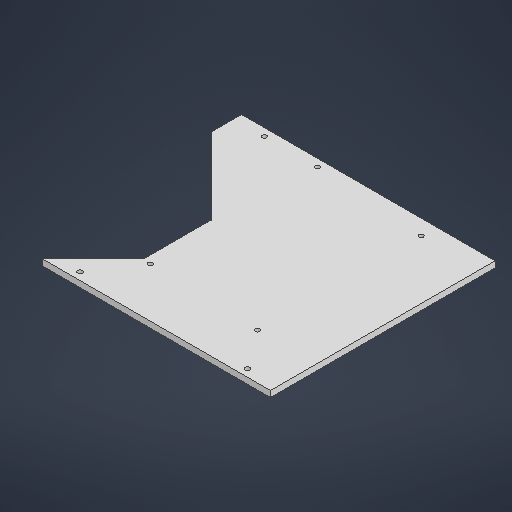
# Autodesk Inventor part: SidePlate_Ebox
Saved by Autodesk Inventor 2025.1 (Build 291241000, 241)
## iProperties
Created: 2025-03-19
Part Number: SidePlate_Ebox
Material: Generic
Document SubType Name: Modeling
Designer: m_kni
Density: 1 g/cm^3
Appearance: Default
Author: m_kni
Autodesk Inventor part; units mm, degrees
ref_plane "YZ Plane" through (0, 0, 0) normal (1, 0, 0) x (0, 1, 0)
ref_plane "XZ Plane" through (0, 0, 0) normal (0, 1, 0) x (-1, 0, 0)
ref_plane "XY Plane" through (0, 0, 0) normal (0, 0, 1) x (1, 0, 0)
sketch "Sketch1" plane through (0, 0, 0) normal (0, 1, 0) x (-1, 0, 0)
  line L0 (-83.0918, 73.8924) -> (-83.0918, -73.6076)
  line L1 (-83.0918, 73.8924) -> (-83.0918, -73.6076)
  line L2 (66.9082, 73.8924) -> (-83.0918, 73.8924)
  line L3 (-83.0918, 73.8924) -> (-83.0918, -73.6076)
  line L4 (-83.0918, -73.6076) -> (83.4082, -73.6076)
  line L5 (83.4082, -73.6076) -> (83.4082, -53.6076)
  line L6 (83.4082, -53.6076) -> (33.4082, -3.6076)
  line L7 (33.4082, -3.6076) -> (33.4082, 40.3924)
  line L8 (33.4082, 40.3924) -> (66.9082, 73.8924)
  point P0 (0, 0)
  point P1 (-8.0918, 73.8924)
  constraints: 18 end point, 1 vertical
extrude "Extrusion1" add sketch "Sketch1" along normal blind 4
sketch "Sketch2" plane through (0, 4, 0) normal (0, 1, 0) x (1, 0, 0)
  line L0 (83.0918, -73.8924) -> (83.0918, 73.6076) projected
  line L1 (-66.9082, -73.8924) -> (83.0918, -73.8924) projected
  line L2 (83.0918, -73.8924) -> (-66.9082, -73.8924)
  circle A0 centre (-46.9082, -68.8924) radius 1.6
  circle A1 centre (63.0918, -68.8924) radius 1.6
  point P0 (0, 0)
  dimension "d2" = 20
  dimension "d3" = 5
  dimension "d4" = 20
  dimension "d5" = 3.2
  dimension "d6" = 3.2
  constraints: 2 centre point, 2 coincident, 2 end point, 1 collinear
  measures "d2" horizontal distance of point (-46.908, -68.892) L1.start
  measures "d3" distance from line of L1 point (-46.908, -68.892)
  measures "d4" distance from line of point (63.092, -68.892) L0
  measures "d5" diameter of A0
  measures "d6" diameter of A1
extrude "Extrusion2" cut sketch "Sketch2" against normal blind 10
sketch "Sketch3" plane through (0, 4, 0) normal (0, 1, 0) x (1, 0, 0)
  line L0 (83.0918, 73.6076) -> (-83.4082, 73.6076) projected
  line L1 (-83.4082, 73.6076) -> (-83.4082, 53.6076) projected
  circle A0 centre (-63.4082, 68.6076) radius 1.5
  circle A1 centre (-28.4082, 68.6076) radius 1.5
  circle A2 centre (-28.4082, -41.3924) radius 1.5
  point P0 (0, 0)
  dimension "d9" = 5
  dimension "d10" = 20
  dimension "d11" = 3
  dimension "d12" = 35
  dimension "d13" = 110
  dimension "d14" = 3
  dimension "d15" = 3
  constraints: 3 centre point, 3 coincident
  measures "d9" distance from line of point (-63.408, 68.608) L0
  measures "d10" distance from line of L1 point (-63.408, 68.608)
  measures "d11" diameter of A0
  measures "d12" distance of point (-28.408, 68.608) A0.centre
  measures "d13" distance of point (-28.408, -41.392) point (-28.408, 68.608)
  measures "d14" diameter of A1
  measures "d15" diameter of A2
extrude "Extrusion3" cut sketch "Sketch3" against normal blind 10
sketch "Sketch4" plane through (0, 4, 0) normal (0, 1, 0) x (1, 0, 0)
  line L0 (83.0918, -73.8924) -> (83.0918, 73.6076) projected
  line L1 (-66.9082, -73.8924) -> (83.0918, -73.8924) projected
  circle A0 centre (44.5918, 63.6076) radius 1.5
  circle A1 centre (44.5918, -43.8924) radius 1.5
  point P0 (0, 0)
  dimension "d18" = 38.5
  dimension "d19" = 30
  dimension "d20" = 107.5
  dimension "d21" = 3
  dimension "d22" = 3
  constraints: 2 centre point, 2 coincident
  measures "d18" distance from line of L0 point (44.592, -43.892)
  measures "d19" distance from line of point (44.592, -43.892) L1
  measures "d20" distance of point (44.592, 63.608) point (44.592, -43.892)
  measures "d21" diameter of A0
  measures "d22" diameter of A1
extrude "Extrusion4" cut sketch "Sketch4" against normal blind 10
body "Solid1"
